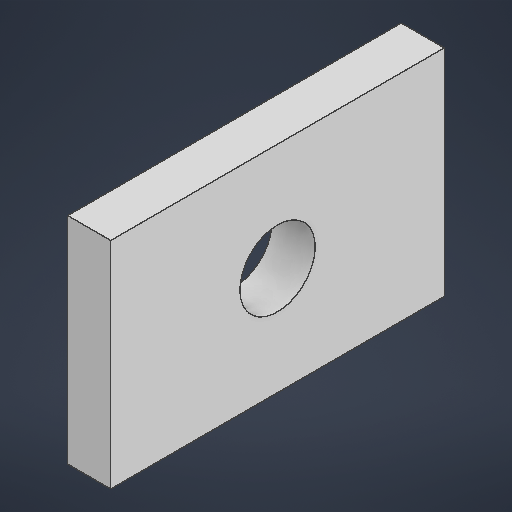
# Autodesk Inventor part: yellow_plate_screw_grip_2
Saved by Autodesk Inventor 2026.1 (Build 301233000, 233)
## iProperties
Created: 2025-10-15
Part Number: yellow_plate_screw_grip_2
Material: Generic
Document SubType Name: Modeling
Designer: emanuel
Density: 1 g/cm^3
Appearance: Default
Author: emanuel
Autodesk Inventor part; units mm, degrees
ref_plane "YZ Plane" through (0, 0, 0) normal (1, 0, 0) x (0, 1, 0)
ref_plane "XZ Plane" through (0, 0, 0) normal (0, 1, 0) x (-1, 0, 0)
ref_plane "XY Plane" through (0, 0, 0) normal (0, 0, 1) x (1, 0, 0)
sketch "Sketch1" plane through (0, 0, 0) normal (1, 0, 0) x (0, 1, 0)
  line L0 (0, 0) -> (10, 0)
  line L1 (10, 0) -> (10, -3.5)
  line L2 (10, -3.5) -> (0, -3.5)
  line L3 (0, -3.5) -> (0, 0)
  line L4 (10, -3.5) -> (0, -3.5)
  line L5 (0, -3.5) -> (0, -6)
  line L6 (0, -6) -> (10, -6)
  line L7 (10, -6) -> (10, -3.5)
  line L8 (10, -6) -> (0, -6)
  line L9 (0, -6) -> (0, -9.5)
  line L10 (0, -9.5) -> (10, -9.5)
  line L11 (10, -9.5) -> (10, -6)
  line L12 (10, -9.5) -> (0, -9.5)
  line L13 (0, -9.5) -> (0, -12)
  line L14 (0, -12) -> (10, -12)
  line L15 (10, -12) -> (10, -9.5)
  line L16 (10, -12) -> (0, -12)
  line L17 (0, -12) -> (0, -15.5)
  line L18 (0, -15.5) -> (10, -15.5)
  line L19 (10, -15.5) -> (10, -12)
  line L20 (10, -7.75) -> (5, -7.75)
  circle A0 centre (5, -7.75) radius 1.75
  line L21 (6.75, -9.5) -> (3.25, -9.5)
  line L22 (3.25, -9.5) -> (3.25, -6)
  line L23 (3.25, -6) -> (6.75, -6)
  line L24 (6.75, -6) -> (6.75, -9.5)
  line L25 (6.75, -9.5) -> (3.25, -6) construction
  line L26 (3.25, -9.5) -> (6.75, -6) construction
  dimension "d0" = 10
  dimension "d1" = 3.5
  dimension "d2" = 2.5
  dimension "d3" = 3.5
  dimension "d4" = 2.5
  dimension "d5" = 3.5
  dimension "d8" = 3.5
  dimension "d11" = 3.5
  constraints: 54 end point, 12 parallel, 7 horizontal, 6 perpendicular, 5 point on line, 3 midpoint, 1 centre point, 1 coincident
  measures "d0" distance of L1.end L2.end
  measures "d1" distance of L0.end L1.end
  measures "d2" distance of L5.end L4.end
  measures "d3" distance of L9.end L8.end
  measures "d4" distance of L13.end L12.end
  measures "d5" distance of L17.end L16.end
  measures "d8" diameter of A0
  measures "d11" distance of L22.end L23.end
extrude "Extrusion1" add sketch "Sketch1" along normal blind 2 contours L0 L1 L2 L3 | L2 L7 L6 L5 | L6 L22 L10 L9 | L11 L20 L24 L6 | L6 A0 L22 | L10 L15 L14 L13 | L24 A0 L6 | L11 L10 L24 L20 | A0 L10 L22 | L14 L19 L18 L17 | L24 L10 A0
body "Solid1"
